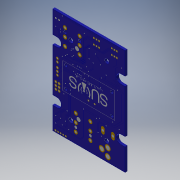
# Autodesk Inventor part: PCB
Saved by Autodesk Inventor 2016 (Build 200138000, 138)
## iProperties
Created: 2015-09-15
Part Number: PCB
Material: Generic
Document SubType Name: Modeling
Designer: Tyler
Density: 1 g/cm^3
Appearance: Smooth - Dark Forest Green
Author: Tyler
Autodesk Inventor part; units mm, degrees
ref_plane "YZ Plane" through (0, 0, 0) normal (1, 0, 0) x (0, 1, 0)
ref_plane "XZ Plane" through (0, 0, 0) normal (0, 1, 0) x (-1, 0, 0)
ref_plane "XY Plane" through (0, 0, 0) normal (0, 0, 1) x (1, 0, 0)
sketch "Sketch1" plane through (0, 0, 0) normal (0, 1, 0) x (-1, 0, 0)
  line L0 (28.305, -41.33) -> (-28.305, -41.33)
  line L1 (-28.305, -41.33) -> (-28.305, 41.33)
  line L2 (-28.305, 41.33) -> (28.305, 41.33)
  line L3 (28.305, 41.33) -> (28.305, -41.33)
  point P0 (0, 0)
  dimension "d0" = 56.61
  dimension "d1" = 82.66
  dimension "d2" = 41.33
  dimension "d3" = 28.305
  constraints: 8 end point, 2 parallel, 1 horizontal, 1 perpendicular
  measures "d0" distance of L0.start L0.end
  measures "d1" distance of L0.end L1.end
  measures "d2" distance from line of point (0, 0) L0
  measures "d3" distance from line of point (0, 0) L1
extrude "Extrusion1" add sketch "Sketch1" along normal blind 1.7
sketch "Sketch2" plane through (0, 1.7, 0) normal (0, 1, 0) x (1, 0, 0)
  line L0 (28.305, 41.33) -> (-28.305, 41.33) projected
  line L1 (28.305, -41.33) -> (28.305, 41.33) projected
  line L2 (25, 20.43) -> (35, 20.43) construction
  line L3 (25, 17.115) -> (35, 17.115)
  line L4 (35, 23.745) -> (25, 23.745)
  arc A0 (25, 23.745) -> (25, 17.115) centre (25, 20.43) ccw
  arc A1 (35, 17.115) -> (35, 23.745) centre (35, 20.43) ccw
  line L5 (0, 0) -> (0, 18.0494) construction
  line L6 (-25, 20.43) -> (-35, 20.43) construction
  line L7 (-25, 17.115) -> (-35, 17.115)
  line L8 (-35, 23.745) -> (-25, 23.745)
  arc A2 (-25, 17.115) -> (-25, 23.745) centre (-25, 20.43) ccw
  arc A3 (-35, 23.745) -> (-35, 17.115) centre (-35, 20.43) ccw
  line L9 (-28.305, -41.33) -> (28.305, -41.33) projected
  line L10 (0, 0) -> (21.685, 0) construction
  line L11 (25, -20.43) -> (35, -20.43) construction
  line L12 (25, -17.115) -> (35, -17.115)
  line L13 (35, -23.745) -> (25, -23.745)
  arc A4 (25, -17.115) -> (25, -23.745) centre (25, -20.43) ccw
  arc A5 (35, -23.745) -> (35, -17.115) centre (35, -20.43) ccw
  line L14 (-25, -20.43) -> (-35, -20.43) construction
  line L15 (-25, -17.115) -> (-35, -17.115)
  line L16 (-35, -23.745) -> (-25, -23.745)
  arc A6 (-25, -23.745) -> (-25, -17.115) centre (-25, -20.43) ccw
  arc A7 (-35, -17.115) -> (-35, -23.745) centre (-35, -20.43) ccw
  point P0 (30, 20.43)
  point P1 (-30, 20.43)
  point P2 (30, -20.43)
  point P3 (-30, -20.43)
  dimension "d6" = 6.63
  dimension "d8" = 6.62
  dimension "d9" = 10
  dimension "d27" = 40.86
  dimension "d28" = 20.9
  dimension "d29" = 20.43
  dimension "d30" = 20.43
  dimension "d31" = 41.33
  dimension "d32" = 41.33
  dimension "d33" = 20.9
  constraints: 36 end point, 21 symmetric about line, 16 point on circle, 8 centre point, 4 tangent, 3 parallel, 1 midpoint, 1 perpendicular, 6 other
  measures "d6" diameter of A1
  measures "d9" distance of L2.start L2.end
  measures "d27" distance between parallel lines of L11 L2
  measures "d28" distance between parallel lines of L9 L11
  measures "d29" distance between parallel lines of L10 L2
  measures "d30" distance between parallel lines of L10 L11
  measures "d31" distance between parallel lines of L9 L10
  measures "d32" distance between parallel lines of L0 L10
  measures "d33" distance between parallel lines of L2 L0
extrude "Extrusion2" cut sketch "Sketch2" against normal through all
sketch "Sketch3" plane through (0, 1.7, 0) normal (0, 1, 0) x (1, 0, 0)
  line L0 (-28.305, 17.115) -> (-28.305, -41.33) projected
  line L1 (-28.305, -41.33) -> (28.305, -41.33) projected
  line L2 (-28.305, 41.33) -> (-28.305, 23.745) projected
  point P0 (0, 0)
  point P1 (-13.995, -27)
  point P2 (14.005, -27)
  point P3 (14.005, 27)
  point P4 (-13.995, 27)
  dimension "d12" = 14.31
  dimension "d13" = 14.33
  dimension "d14" = 28
  dimension "d15" = 28
  dimension "d16" = 54
  dimension "d17" = 14.33
  dimension "d18" = 14.31
  dimension "d19" = 54
  measures "d12" distance from line of L0 point (-13.995, -27)
  measures "d13" distance from line of L1 point (-13.995, -27)
  measures "d14" distance of point (-13.995, -27) point (14.005, -27)
  measures "d15" distance of point (14.005, 27) point (-13.995, 27)
  measures "d16" distance of point (-13.995, -27) point (-13.995, 27)
  measures "d17" distance from line of L1 point (14.005, -27)
  measures "d18" distance from line of L2 point (-13.995, 27)
  measures "d19" distance of point (14.005, -27) point (14.005, 27)
hole "Hole1" at (-13.995, 1.7, 27) at (14.005, 1.7, 27) at (14.005, 1.7, -27) at (-13.995, 1.7, -27) direction (0, -1, 0) diameter 3.2 end through all
sketch "Sketch4" plane through (0, 1.7, 0) normal (0, 1, 0) x (1, 0, 0)
  line L0 (-28.305, -41.33) -> (28.305, -41.33) projected
  line L1 (28.305, 41.33) -> (-28.305, 41.33) projected
  line L2 (-28.305, 17.115) -> (-28.305, -17.115) projected
  line L3 (18, -8) -> (-18, -8) construction
  line L4 (-18, -8) -> (-18, 8) construction
  line L5 (-18, 8) -> (18, 8) construction
  line L6 (18, 8) -> (18, -8) construction
  line L7 (18, -8) -> (-18, 8) construction
  line L8 (-18, -8) -> (18, 8) construction
  point P0 (0, 0)
  point P1 (0, 0)
  dimension "d34" = 36
  dimension "d35" = 16
  dimension "d36" = 28.305
  dimension "d37" = 56.61
  dimension "d38" = 82.66
  dimension "d39" = 41.33
  constraints: 12 end point, 4 coincident, 2 midpoint, 2 parallel, 1 horizontal, 1 perpendicular
  measures "d34" distance of L4.end L5.end
  measures "d35" distance of L3.end L4.end
  measures "d36" distance from line of L2 point (0, 0)
  measures "d37" distance of L1.start L1.end
  measures "d38" distance between parallel lines of L0 L1
  measures "d39" distance from line of point (0, 0) L1
hole "Hole2" at (-18, 1.7, -8) at (-18, 1.7, 8) at (18, 1.7, 8) at (18, 1.7, -8) direction (0, -1, 0) diameter 2 end through all
sketch "Sketch5" plane through (0, 1.7, 0) normal (0, 1, 0) x (1, 0, 0)
  line L0 (-28.305, -23.745) -> (-28.305, -41.33) projected
  line L1 (-28.305, -41.33) -> (28.305, -41.33) projected
  circle A0 centre (-18.535, -30.07) radius 1
  circle A1 centre (-7.105, -30.07) radius 1
  point P0 (0, 0)
  dimension "d47" = 9.77
  dimension "d48" = 11.26
  dimension "d49" = 21.2
  dimension "d50" = 11.26
  dimension "d51" = 2
  dimension "d52" = 2
  dimension "d53" = 11.43
  constraints: 2 centre point
  measures "d47" distance from line of L0 A0.centre
  measures "d48" distance from line of L1 A0.centre
  measures "d49" distance from line of L0 A1.centre
  measures "d50" distance from line of L1 A1.centre
  measures "d51" diameter of A0
  measures "d52" diameter of A1
  measures "d53" distance of A1.centre A0.centre
extrude "Extrusion3" cut sketch "Sketch5" against normal through all
sketch "Sketch6" plane through (0, 1.7, 0) normal (0, 1, 0) x (1, 0, 0)
  line L0 (-28.352, 41.33) -> (28.305, 41.33) construction
  line L1 (28.305, 41.33) -> (28.305, -41.33) construction
  line L2 (28.305, -41.33) -> (-28.352, -41.33) construction
  line L3 (-28.352, -41.33) -> (-28.352, 41.33) construction
  line L4 (28.305, 41.33) -> (-28.305, 41.33) projected
  line L5 (-28.305, -41.33) -> (28.305, -41.33) projected
  line L6 (28.305, -17.115) -> (28.305, 17.115) projected
  point P0 (0, 0)
  constraints: 3 collinear, 2 other
decal "Decal1"
sketch "Sketch7" plane through (0, 0, 0) normal (0, -1, 0) x (1, 0, 0)
  line L0 (-28.352, 41.33) -> (28.305, 41.33) construction
  line L1 (28.305, 41.33) -> (28.305, -41.33) construction
  line L2 (28.305, -41.33) -> (-28.352, -41.33) construction
  line L3 (-28.352, -41.33) -> (-28.352, 41.33) construction
  line L4 (28.305, 41.33) -> (-28.305, 41.33) projected
  line L5 (-28.305, -41.33) -> (28.305, -41.33) projected
  line L6 (28.305, -17.115) -> (28.305, 17.115) projected
  point P0 (0, 0)
  constraints: 3 collinear, 2 other
decal "Decal2"
equation "\"d2\" = 0.5 * d1"
equation "\"d3\" = 0.5 * d0"
equation "\"d17\" = d13"
equation "\"d18\" = d12"
equation "\"d19\" = d16"
equation "\"d36\" = 0.5 * d37"
equation "\"d39\" = 0.5 * d38"
equation "\"d52\" = d51"
body "Solid1"
